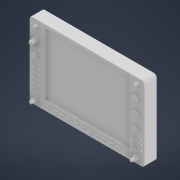
# Autodesk Inventor part: G1000
Saved by Autodesk Inventor 2022 (Build 260153000, 153)
## iProperties
Created: 2022-01-12
Part Number: G1000
Material: Generic
Document SubType Name: Modeling
Designer: diabolous
Density: 1 g/cm^3
Appearance: Default
Author: diabolous
Autodesk Inventor part; units mm, degrees
ref_plane "YZ Plane" through (0, 0, 0) normal (1, 0, 0) x (0, 1, 0)
ref_plane "XZ Plane" through (0, 0, 0) normal (0, 1, 0) x (-1, 0, 0)
ref_plane "XY Plane" through (0, 0, 0) normal (0, 0, 1) x (1, 0, 0)
sketch "Sketch2" plane through (0, 0, 0) normal (0, 0, 1) x (1, 0, 0)
  line L0 (0, 0) -> (296.2402, 0)
  line L1 (296.2402, 0) -> (296.2402, 193.548)
  line L2 (296.2402, 193.548) -> (0, 193.548)
  line L3 (0, 193.548) -> (0, 0)
  dimension "d29" = 296.2402
  dimension "d30" = 193.548
  constraints: 8 end point, 2 parallel, 1 horizontal, 1 perpendicular
  measures "d29" distance of L2.end L1.end
  measures "d30" distance of L1.end L0.end
extrude "Extrusion1" add sketch "Sketch2" along normal blind 32.3
fillet "Fillet1" radius 7.9375 4 edges at (296.2402, 193.548, 16.15) (296.2402, 0, 16.15) (0, 0, 16.15) (0, 193.548, 16.15)
sketch "Sketch3" plane through (0, 0, 32.3) normal (0, 0, 1) x (1, 0, 0)
  line L0 (7.9375, 0) -> (288.3027, 0) projected
  line L1 (296.2402, 7.9375) -> (296.2402, 185.6105) projected
  line L2 (288.3027, 193.548) -> (7.9375, 193.548) projected
  line L3 (0, 185.6105) -> (0, 7.9375) projected
  line L4 (0, 185.6105) -> (0, 7.9375) projected
  line L5 (40.7162, 183.3372) -> (255.524, 183.3372)
  line L6 (255.524, 183.3372) -> (255.524, 22.987)
  line L7 (255.524, 22.987) -> (40.7162, 22.987)
  line L8 (40.7162, 22.987) -> (40.7162, 183.3372)
  point P0 (0, 0)
  point P1 (40.7162, 0)
  point P2 (255.524, 0)
  point P3 (296.2402, 183.3372)
  point P4 (255.524, 193.548)
  point P5 (40.7162, 193.548)
  point P6 (0, 22.987)
  point P7 (296.2402, 22.987)
  point P8 (0, 183.3372)
  dimension "d34" = 40.7162
  dimension "d35" = 40.7162
  dimension "d36" = 10.2108
  dimension "d37" = 40.7162
  dimension "d38" = 22.987
  dimension "d39" = 22.987
  dimension "d40" = 40.7162
  dimension "d41" = 10.2108
  constraints: 8 end point, 6 point on line, 2 parallel, 1 horizontal, 1 perpendicular
  measures "d34" distance of point (40.716, 0) point (0, 0)
  measures "d35" distance from line of L1 point (255.524, 193.548)
  measures "d36" distance from line of L2 point (296.24, 183.337)
  measures "d37" distance from line of L1 point (255.524, 0)
  measures "d38" distance from line of L0 point (296.24, 22.987)
  measures "d39" distance from line of point (0, 22.987) L0
  measures "d40" distance from line of L3 point (40.716, 193.548)
  measures "d41" distance from line of L2 point (0, 183.337)
extrude "Extrusion2" cut sketch "Sketch3" against normal blind 5.08
sketch "Sketch4" plane through (0, 0, 32.3) normal (0, 0, 1) x (1, 0, 0)
  line L0 (288.3027, 193.548) -> (7.9375, 193.548) projected
  line L1 (296.2402, 7.9375) -> (296.2402, 185.6105) projected
  line L2 (0, 185.6105) -> (0, 7.9375) projected
  circle A0 centre (18.5928, 178.5874) radius 3.9243
  circle A1 centre (277.6474, 178.5874) radius 3.9243
  point P0 (0, 0)
  point P1 (0, 178.5874)
  point P2 (18.5928, 193.548)
  point P3 (277.6474, 193.548)
  point P4 (296.2402, 178.5874)
  dimension "d44" = 14.9606
  dimension "d45" = 14.9606
  dimension "d46" = 18.5928
  dimension "d47" = 18.5928
  dimension "d48" = 7.8486
  constraints: 3 point on line, 2 centre point
  measures "d44" distance from line of L0 point (0, 178.587)
  measures "d45" distance from line of L0 point (296.24, 178.587)
  measures "d46" distance from line of L2 point (18.593, 193.548)
  measures "d47" distance from line of L1 point (277.647, 193.548)
  measures "d48" diameter of A0
extrude "Extrusion3" add sketch "Sketch4" along normal blind 8.255
sketch "Sketch5" plane through (0, 0, 32.3) normal (0, 0, 1) x (1, 0, 0)
  circle A0 centre (18.5928, 178.5874) radius 3.9243 projected
  line L0 (18.5928, 178.5874) -> (18.5928, 0) construction
  line L1 (7.9375, 0) -> (288.3027, 0) projected
  line L2 (0, 185.6105) -> (0, 7.9375) projected
  line L3 (288.3027, 193.548) -> (7.9375, 193.548) projected
  circle A1 centre (18.5928, 149.3012) radius 6.1341
  circle A2 centre (18.5928, 115.2144) radius 6.1849
  circle A3 centre (18.5928, 15.9766) radius 6.096
  point P0 (0, 0)
  point P1 (0, 149.3012)
  point P2 (0, 115.2144)
  point P3 (0, 15.9766)
  dimension "d51" = 44.2468
  dimension "d52" = 78.3336
  dimension "d53" = 177.5714
  dimension "d54" = 12.2682
  dimension "d55" = 12.3698
  dimension "d56" = 12.192
  constraints: 7 point on line, 3 centre point, 2 end point, 1 vertical
  measures "d51" distance from line of point (0, 149.301) L3
  measures "d52" distance from line of L3 point (0, 115.214)
  measures "d53" distance from line of L3 point (0, 15.977)
  measures "d54" diameter of A1
  measures "d55" diameter of A2
  measures "d56" diameter of A3
extrude "Extrusion4" add sketch "Sketch5" along normal blind 8.255 contours A1 | A2 | A3
sketch "Sketch6" plane through (18.5928, 115.2144, 40.555) normal (0, 0, 1) x (1, 0, 0)
  circle A0 centre (0, 34.0868) radius 6.1341 projected
  circle A1 centre (0, 34.0868) radius 4.8387
  circle A2 centre (0, -99.2378) radius 6.096 projected
  circle A3 centre (0, -99.2378) radius 3.9751
  point P0 (-18.5928, -115.2144)
  dimension "d59" = 9.6774
  dimension "d60" = 7.9502
  constraints: 2 centre point, 2 coincident
  measures "d59" diameter of A1
  measures "d60" diameter of A3
extrude "Extrusion5" add sketch "Sketch6" along normal blind 8.255 contours A1 | A3
sketch "Sketch7" plane through (0, 0, 32.3) normal (0, 0, 1) x (1, 0, 0)
  line L0 (7.9375, 0) -> (288.3027, 0) projected
  line L1 (40.7162, 11.9126) -> (255.524, 11.9126) construction
  line L2 (148.1201, 0) -> (148.1201, 193.548) construction
  line L3 (288.3027, 193.548) -> (7.9375, 193.548) projected
  line L4 (54.2163, 9.3726) -> (44.0563, 9.3726)
  line L5 (44.0563, 9.3726) -> (44.0563, 14.4526)
  line L6 (44.0563, 14.4526) -> (54.2163, 14.4526)
  line L7 (54.2163, 14.4526) -> (54.2163, 9.3726)
  line L8 (54.2163, 9.3726) -> (44.0563, 14.4526) construction
  line L9 (44.0563, 9.3726) -> (54.2163, 14.4526) construction
  line L10 (72.1487, 9.3726) -> (61.9887, 9.3726)
  line L11 (61.9887, 9.3726) -> (61.9887, 14.4526)
  line L12 (61.9887, 14.4526) -> (72.1487, 14.4526)
  line L13 (72.1487, 14.4526) -> (72.1487, 9.3726)
  line L14 (72.1487, 9.3726) -> (61.9887, 14.4526) construction
  line L15 (61.9887, 9.3726) -> (72.1487, 14.4526) construction
  line L16 (90.0811, 9.3726) -> (79.9211, 9.3726)
  line L17 (79.9211, 9.3726) -> (79.9211, 14.4526)
  line L18 (79.9211, 14.4526) -> (90.0811, 14.4526)
  line L19 (90.0811, 14.4526) -> (90.0811, 9.3726)
  line L20 (90.0811, 9.3726) -> (79.9211, 14.4526) construction
  line L21 (79.9211, 9.3726) -> (90.0811, 14.4526) construction
  line L22 (108.0135, 9.3726) -> (97.8535, 9.3726)
  line L23 (97.8535, 9.3726) -> (97.8535, 14.4526)
  line L24 (97.8535, 14.4526) -> (108.0135, 14.4526)
  line L25 (108.0135, 14.4526) -> (108.0135, 9.3726)
  line L26 (108.0135, 9.3726) -> (97.8535, 14.4526) construction
  line L27 (97.8535, 9.3726) -> (108.0135, 14.4526) construction
  line L28 (125.9459, 9.3726) -> (115.7859, 9.3726)
  line L29 (115.7859, 9.3726) -> (115.7859, 14.4526)
  line L30 (115.7859, 14.4526) -> (125.9459, 14.4526)
  line L31 (125.9459, 14.4526) -> (125.9459, 9.3726)
  line L32 (125.9459, 9.3726) -> (115.7859, 14.4526) construction
  line L33 (115.7859, 9.3726) -> (125.9459, 14.4526) construction
  line L34 (143.8783, 9.3726) -> (133.7183, 9.3726)
  line L35 (133.7183, 9.3726) -> (133.7183, 14.4526)
  line L36 (133.7183, 14.4526) -> (143.8783, 14.4526)
  line L37 (143.8783, 14.4526) -> (143.8783, 9.3726)
  line L38 (143.8783, 9.3726) -> (133.7183, 14.4526) construction
  line L39 (133.7183, 9.3726) -> (143.8783, 14.4526) construction
  line L40 (162.5219, 9.3726) -> (152.3619, 9.3726)
  line L41 (152.3619, 9.3726) -> (152.3619, 14.4526)
  line L42 (152.3619, 14.4526) -> (162.5219, 14.4526)
  line L43 (162.5219, 14.4526) -> (162.5219, 9.3726)
  line L44 (162.5219, 9.3726) -> (152.3619, 14.4526) construction
  line L45 (152.3619, 9.3726) -> (162.5219, 14.4526) construction
  line L46 (180.4543, 9.3726) -> (170.2943, 9.3726)
  line L47 (170.2943, 9.3726) -> (170.2943, 14.4526)
  line L48 (170.2943, 14.4526) -> (180.4543, 14.4526)
  line L49 (180.4543, 14.4526) -> (180.4543, 9.3726)
  line L50 (180.4543, 9.3726) -> (170.2943, 14.4526) construction
  line L51 (170.2943, 9.3726) -> (180.4543, 14.4526) construction
  line L52 (198.3867, 9.3726) -> (188.2267, 9.3726)
  line L53 (188.2267, 9.3726) -> (188.2267, 14.4526)
  line L54 (188.2267, 14.4526) -> (198.3867, 14.4526)
  line L55 (198.3867, 14.4526) -> (198.3867, 9.3726)
  line L56 (198.3867, 9.3726) -> (188.2267, 14.4526) construction
  line L57 (188.2267, 9.3726) -> (198.3867, 14.4526) construction
  line L58 (216.3191, 9.3726) -> (206.1591, 9.3726)
  line L59 (206.1591, 9.3726) -> (206.1591, 14.4526)
  line L60 (206.1591, 14.4526) -> (216.3191, 14.4526)
  line L61 (216.3191, 14.4526) -> (216.3191, 9.3726)
  line L62 (216.3191, 9.3726) -> (206.1591, 14.4526) construction
  line L63 (206.1591, 9.3726) -> (216.3191, 14.4526) construction
  line L64 (234.2515, 9.3726) -> (224.0915, 9.3726)
  line L65 (224.0915, 9.3726) -> (224.0915, 14.4526)
  line L66 (224.0915, 14.4526) -> (234.2515, 14.4526)
  line L67 (234.2515, 14.4526) -> (234.2515, 9.3726)
  line L68 (234.2515, 9.3726) -> (224.0915, 14.4526) construction
  line L69 (224.0915, 9.3726) -> (234.2515, 14.4526) construction
  line L70 (252.1839, 9.3726) -> (242.0239, 9.3726)
  line L71 (242.0239, 9.3726) -> (242.0239, 14.4526)
  line L72 (242.0239, 14.4526) -> (252.1839, 14.4526)
  line L73 (252.1839, 14.4526) -> (252.1839, 9.3726)
  line L74 (252.1839, 9.3726) -> (242.0239, 14.4526) construction
  line L75 (242.0239, 9.3726) -> (252.1839, 14.4526) construction
  point P0 (0, 0)
  point P1 (138.7983, 11.9126)
  point P2 (120.8659, 11.9126)
  point P3 (102.9335, 11.9126)
  point P4 (85.0011, 11.9126)
  point P5 (67.0687, 11.9126)
  point P6 (49.1363, 11.9126)
  point P7 (157.4419, 11.9126)
  point P8 (175.3743, 11.9126)
  point P9 (193.3067, 11.9126)
  point P10 (211.2391, 11.9126)
  point P11 (229.1715, 11.9126)
  point P12 (247.1039, 11.9126)
  dimension "d63" = 11.9126
  dimension "d64" = 11.9126
  dimension "d65" = 9.3218
  dimension "d66" = 17.9324
  dimension "d67" = 17.9324
  dimension "d68" = 17.9324
  dimension "d69" = 17.9324
  dimension "d70" = 17.9324
  dimension "d71" = 9.3218
  dimension "d72" = 17.9324
  dimension "d73" = 17.9324
  dimension "d74" = 17.9324
  dimension "d75" = 17.9324
  dimension "d76" = 17.9324
  dimension "d77" = 10.16
  dimension "d78" = 5.08
  dimension "d79" = 10.16
  dimension "d80" = 10.16
  dimension "d81" = 10.16
  dimension "d82" = 10.16
  dimension "d83" = 10.16
  dimension "d84" = 10.16
  dimension "d85" = 10.16
  dimension "d86" = 10.16
  dimension "d87" = 10.16
  dimension "d88" = 10.16
  dimension "d89" = 10.16
  constraints: 146 end point, 26 midpoint, 24 parallel, 12 horizontal, 12 perpendicular, 11 point on line, 15 other
  measures "d63" distance from line of L0 point (40.716, 11.913)
  measures "d64" distance from line of L0 point (255.524, 11.913)
  measures "d65" distance from line of L2 point (138.798, 11.913)
  measures "d66" distance of point (138.798, 11.913) point (120.866, 11.913)
  measures "d67" distance of point (102.934, 11.913) point (120.866, 11.913)
  measures "d68" distance of point (85.001, 11.913) point (102.934, 11.913)
  measures "d69" distance of point (67.069, 11.913) point (85.001, 11.913)
  measures "d70" distance of point (49.136, 11.913) point (67.069, 11.913)
  measures "d71" distance from line of point (157.442, 11.913) L2
  measures "d72" distance of point (175.374, 11.913) point (157.442, 11.913)
  measures "d73" distance of point (193.307, 11.913) point (175.374, 11.913)
  measures "d74" distance of point (211.239, 11.913) point (193.307, 11.913)
  measures "d75" distance of point (229.172, 11.913) point (211.239, 11.913)
  measures "d76" distance of point (247.104, 11.913) point (229.172, 11.913)
  measures "d77" distance of L5.end L6.end
  measures "d78" distance of L4.end L5.end
  measures "d79" distance of L11.end L12.end
  measures "d80" distance of L17.end L18.end
  measures "d81" distance of L23.end L24.end
  measures "d82" distance of L29.end L30.end
  measures "d83" distance of L35.end L36.end
  measures "d84" distance of L41.end L42.end
  measures "d85" distance of L47.end L48.end
  measures "d86" distance of L53.end L54.end
  measures "d87" distance of L59.end L60.end
  measures "d88" distance of L65.end L66.end
  measures "d89" distance of L71.end L72.end
extrude "Extrusion6" add sketch "Sketch7" along normal blind 1.905
fillet "Fillet2" radius 2.54 1 edges at (14.6685, 178.5874, 32.3)
fillet "Fillet3" radius 2.54 4 edges at (12.4587, 149.3012, 32.3) (12.4079, 115.2144, 32.3) (12.4968, 15.9766, 32.3) (273.7231, 178.5874, 32.3)
fillet "Fillet4" radius 2.54 8 edges at (40.7162, 103.1621, 27.22) (148.1201, 22.987, 27.22) (148.1201, 183.3372, 27.22) (255.524, 103.1621, 27.22) (40.7162, 103.1621, 32.3) (148.1201, 22.987, 32.3) (148.1201, 183.3372, 32.3) (255.524, 103.1621, 32.3)
fillet "Fillet5" radius 0.9525 23 edges at (14.6685, 178.5874, 40.555) (12.4587, 149.3012, 40.555) (13.7541, 149.3012, 48.81) (12.4079, 115.2144, 40.555) (14.6177, 15.9766, 48.81) (12.4968, 15.9766, 40.555) (293.9154, 2.3248, 32.3) (296.2402, 96.774, 32.3) (293.9154, 191.2232, 32.3) (148.1201, 193.548, 32.3) (2.3248, 191.2232, 32.3) (0, 96.774, 32.3) (2.3248, 2.3248, 32.3) (148.1201, 0, 32.3) (273.7231, 178.5874, 40.555) (293.9154, 191.2232, 0) (148.1201, 193.548, 0) (2.3248, 191.2232, 0) (0, 96.774, 0) (2.3248, 2.3248, 0) (148.1201, 0, 0) (293.9154, 2.3248, 0) (296.2402, 96.774, 0)
sketch "Sketch8" plane through (0, 0, 32.3) normal (0, 0, 1) x (1, 0, 0)
  circle A0 centre (277.6474, 178.5874) radius 3.9243 projected
  line L0 (277.6474, 178.5874) -> (277.6474, -3.1455)
  line L1 (288.3027, 193.548) -> (7.9375, 193.548) projected
  circle A1 centre (277.6474, 149.3012) radius 6.1341
  circle A2 centre (277.6474, 115.2144) radius 6.1849
  point P0 (0, 0)
  dimension "d96" = 44.2468
  dimension "d97" = 12.2682
  dimension "d98" = 78.3336
  dimension "d99" = 12.3698
  constraints: 2 centre point, 2 coincident, 2 end point, 2 point on line, 1 vertical
  measures "d96" distance from line of point (277.647, 149.301) L1
  measures "d97" diameter of A1
  measures "d98" distance from line of point (277.647, 115.214) L1
  measures "d99" diameter of A2
extrude "Extrusion7" add sketch "Sketch8" along normal blind 8.255 contours A1 L0 | L0 A1 | A2 L0 | L0 A2
fillet "Fillet6" radius 0.9525 2 edges at (271.5133, 149.3012, 40.555) (271.4625, 115.2144, 40.555)
sketch "Sketch9" plane through (0, 0, 32.3) normal (0, 0, 1) x (1, 0, 0)
  circle A0 centre (18.5928, 15.9766) radius 3.0226 projected
  circle A1 centre (277.6474, 115.2144) radius 5.2324 projected
  circle A2 centre (277.6474, 15.9766) radius 6.096
  point P0 (0, 0)
  dimension "d103" = 12.192
  constraints: 1 centre point
  measures "d103" diameter of A2
extrude "Extrusion8" add sketch "Sketch9" along normal blind 8.255 contours A2
sketch "Sketch10" plane through (277.6474, 15.9766, 40.555) normal (0, 0, 1) x (1, 0, 0)
  circle A0 centre (0, 0) radius 6.096 projected
  circle A1 centre (0, 0) radius 3.9751
  point P0 (-277.6474, -15.9766)
  dimension "d106" = 7.9502
  constraints: 1 centre point, 1 coincident
  measures "d106" diameter of A1
extrude "Extrusion9" add sketch "Sketch10" along normal blind 8.255 contours A1
sketch "Sketch11" plane through (0, 0, 32.3) normal (0, 0, 1) x (1, 0, 0)
  line L0 (296.2402, 7.9375) -> (296.2402, 185.6105) projected
  line L1 (288.3027, 0.9525) -> (7.9375, 0.9525) projected
  line L2 (295.2877, 185.6105) -> (295.2877, 7.9375) projected
  line L3 (7.9375, 0) -> (288.3027, 0) projected
  line L4 (269.9512, 0) -> (269.9512, 58.6486) construction
  line L5 (284.6578, 0.9525) -> (284.6578, 58.6486) construction
  line L6 (284.6578, 35.9918) -> (269.9512, 35.9918) construction
  line L7 (284.6578, 47.3202) -> (269.9512, 47.3202) construction
  line L8 (284.6578, 58.6486) -> (269.9512, 58.6486) construction
  line L9 (264.8712, 38.5318) -> (275.0312, 38.5318)
  line L10 (275.0312, 38.5318) -> (275.0312, 33.4518)
  line L11 (275.0312, 33.4518) -> (264.8712, 33.4518)
  line L12 (264.8712, 33.4518) -> (264.8712, 38.5318)
  line L13 (264.8712, 38.5318) -> (275.0312, 33.4518) construction
  line L14 (275.0312, 38.5318) -> (264.8712, 33.4518) construction
  line L15 (289.7378, 33.4518) -> (279.5778, 33.4518)
  line L16 (279.5778, 33.4518) -> (279.5778, 38.5318)
  line L17 (279.5778, 38.5318) -> (289.7378, 38.5318)
  line L18 (289.7378, 38.5318) -> (289.7378, 33.4518)
  line L19 (289.7378, 33.4518) -> (279.5778, 38.5318) construction
  line L20 (279.5778, 33.4518) -> (289.7378, 38.5318) construction
  line L21 (264.8712, 49.8602) -> (275.0312, 49.8602)
  line L22 (275.0312, 49.8602) -> (275.0312, 44.7802)
  line L23 (275.0312, 44.7802) -> (264.8712, 44.7802)
  line L24 (264.8712, 44.7802) -> (264.8712, 49.8602)
  line L25 (264.8712, 49.8602) -> (275.0312, 44.7802) construction
  line L26 (275.0312, 49.8602) -> (264.8712, 44.7802) construction
  line L27 (289.7378, 44.7802) -> (279.5778, 44.7802)
  line L28 (279.5778, 44.7802) -> (279.5778, 49.8602)
  line L29 (279.5778, 49.8602) -> (289.7378, 49.8602)
  line L30 (289.7378, 49.8602) -> (289.7378, 44.7802)
  line L31 (289.7378, 44.7802) -> (279.5778, 49.8602) construction
  line L32 (279.5778, 44.7802) -> (289.7378, 49.8602) construction
  line L33 (264.8712, 61.1886) -> (275.0312, 61.1886)
  line L34 (275.0312, 61.1886) -> (275.0312, 56.1086)
  line L35 (275.0312, 56.1086) -> (264.8712, 56.1086)
  line L36 (264.8712, 56.1086) -> (264.8712, 61.1886)
  line L37 (264.8712, 61.1886) -> (275.0312, 56.1086) construction
  line L38 (275.0312, 61.1886) -> (264.8712, 56.1086) construction
  line L39 (289.7378, 61.1886) -> (279.5778, 61.1886)
  line L40 (279.5778, 61.1886) -> (279.5778, 56.1086)
  line L41 (279.5778, 56.1086) -> (289.7378, 56.1086)
  line L42 (289.7378, 56.1086) -> (289.7378, 61.1886)
  line L43 (289.7378, 61.1886) -> (279.5778, 56.1086) construction
  line L44 (279.5778, 61.1886) -> (289.7378, 56.1086) construction
  point P0 (0, 0)
  point P1 (295.2877, 35.9918)
  point P2 (295.2877, 47.3202)
  point P3 (295.2877, 58.6486)
  dimension "d109" = 26.289
  dimension "d110" = 11.5824
  dimension "d111" = 35.9918
  dimension "d112" = 47.3202
  dimension "d113" = 58.6486
  dimension "d114" = 10.16
  dimension "d115" = 5.08
  dimension "d116" = 10.16
  dimension "d117" = 5.08
  dimension "d118" = 5.08
  constraints: 82 end point, 15 point on line, 14 parallel, 12 midpoint, 8 perpendicular, 6 horizontal, 1 vertical
  measures "d109" distance from line of L0 L4.start
  measures "d110" distance from line of L0 L5.start
  measures "d111" distance from line of point (295.288, 35.992) L3
  measures "d112" distance from line of L3 point (295.288, 47.32)
  measures "d113" distance from line of point (295.288, 58.649) L3
  measures "d114" distance of L10.end L11.end
  measures "d115" distance of L9.end L10.end
  measures "d116" distance of L16.end L17.end
  measures "d117" distance of L21.end L22.end
  measures "d118" distance of L33.end L34.end
extrude "Extrusion10" add sketch "Sketch11" along normal blind 1.905
sketch "Sketch12" plane through (0, 0, 32.3) normal (0, 0, 1) x (1, 0, 0)
  circle A0 centre (277.6474, 115.2144) radius 5.2324 projected
  line L0 (288.3027, 193.548) -> (7.9375, 193.548) projected
  circle A1 centre (277.6474, 81.788) radius 4.6482
  point P0 (0, 0)
  dimension "d121" = 111.76
  dimension "d122" = 9.2964
  constraints: 1 centre point, 1 coincident
  measures "d121" distance from line of point (277.647, 81.788) L0
  measures "d122" diameter of A1
extrude "Extrusion11" add sketch "Sketch12" along normal blind 8.255 contours A1
fillet "Fillet7" radius 0.9525 1 edges at (272.9992, 81.788, 40.555)
sketch "Sketch13" plane through (0, 0, 32.3) normal (0, 0, 1) x (1, 0, 0)
  line L0 (264.8712, 56.1086) -> (264.8712, 61.1886) projected
  line L1 (0.9525, 7.9375) -> (0.9525, 185.6105) projected
  line L2 (264.8712, 44.7802) -> (264.8712, 49.8602) projected
  line L3 (264.8712, 33.4518) -> (264.8712, 38.5318) projected
  line L4 (288.3027, 0.9525) -> (7.9375, 0.9525) projected
  line L5 (0, 185.6105) -> (0, 7.9375) projected
  line L6 (16.6624, 33.4518) -> (6.5024, 33.4518)
  line L7 (6.5024, 33.4518) -> (6.5024, 38.5318)
  line L8 (6.5024, 38.5318) -> (16.6624, 38.5318)
  line L9 (16.6624, 38.5318) -> (16.6624, 33.4518)
  line L10 (16.6624, 33.4518) -> (6.5024, 38.5318) construction
  line L11 (6.5024, 33.4518) -> (16.6624, 38.5318) construction
  line L12 (31.369, 33.4518) -> (21.209, 33.4518)
  line L13 (21.209, 33.4518) -> (21.209, 38.5318)
  line L14 (21.209, 38.5318) -> (31.369, 38.5318)
  line L15 (31.369, 38.5318) -> (31.369, 33.4518)
  line L16 (31.369, 33.4518) -> (21.209, 38.5318) construction
  line L17 (21.209, 33.4518) -> (31.369, 38.5318) construction
  line L18 (16.6624, 44.7802) -> (6.5024, 44.7802)
  line L19 (6.5024, 44.7802) -> (6.5024, 49.8602)
  line L20 (6.5024, 49.8602) -> (16.6624, 49.8602)
  line L21 (16.6624, 49.8602) -> (16.6624, 44.7802)
  line L22 (16.6624, 44.7802) -> (6.5024, 49.8602) construction
  line L23 (6.5024, 44.7802) -> (16.6624, 49.8602) construction
  line L24 (31.369, 44.7802) -> (21.209, 44.7802)
  line L25 (21.209, 44.7802) -> (21.209, 49.8602)
  line L26 (21.209, 49.8602) -> (31.369, 49.8602)
  line L27 (31.369, 49.8602) -> (31.369, 44.7802)
  line L28 (31.369, 44.7802) -> (21.209, 49.8602) construction
  line L29 (21.209, 44.7802) -> (31.369, 49.8602) construction
  line L30 (16.6624, 56.1086) -> (6.5024, 56.1086)
  line L31 (6.5024, 56.1086) -> (6.5024, 61.1886)
  line L32 (6.5024, 61.1886) -> (16.6624, 61.1886)
  line L33 (16.6624, 61.1886) -> (16.6624, 56.1086)
  line L34 (16.6624, 56.1086) -> (6.5024, 61.1886) construction
  line L35 (6.5024, 56.1086) -> (16.6624, 61.1886) construction
  line L36 (31.369, 56.1086) -> (21.209, 56.1086)
  line L37 (21.209, 56.1086) -> (21.209, 61.1886)
  line L38 (21.209, 61.1886) -> (31.369, 61.1886)
  line L39 (31.369, 61.1886) -> (31.369, 56.1086)
  line L40 (31.369, 56.1086) -> (21.209, 61.1886) construction
  line L41 (21.209, 56.1086) -> (31.369, 61.1886) construction
  line L42 (16.6624, 67.437) -> (6.5024, 67.437)
  line L43 (6.5024, 67.437) -> (6.5024, 72.517)
  line L44 (6.5024, 72.517) -> (16.6624, 72.517)
  line L45 (16.6624, 72.517) -> (16.6624, 67.437)
  line L46 (16.6624, 67.437) -> (6.5024, 72.517) construction
  line L47 (6.5024, 67.437) -> (16.6624, 72.517) construction
  line L48 (31.369, 67.437) -> (21.209, 67.437)
  line L49 (21.209, 67.437) -> (21.209, 72.517)
  line L50 (21.209, 72.517) -> (31.369, 72.517)
  line L51 (31.369, 72.517) -> (31.369, 67.437)
  line L52 (31.369, 67.437) -> (21.209, 72.517) construction
  line L53 (21.209, 67.437) -> (31.369, 72.517) construction
  line L54 (16.6624, 78.7654) -> (6.5024, 78.7654)
  line L55 (6.5024, 78.7654) -> (6.5024, 83.8454)
  line L56 (6.5024, 83.8454) -> (16.6624, 83.8454)
  line L57 (16.6624, 83.8454) -> (16.6624, 78.7654)
  line L58 (16.6624, 78.7654) -> (6.5024, 83.8454) construction
  line L59 (6.5024, 78.7654) -> (16.6624, 83.8454) construction
  line L60 (31.369, 78.7654) -> (21.209, 78.7654)
  line L61 (21.209, 78.7654) -> (21.209, 83.8454)
  line L62 (21.209, 83.8454) -> (31.369, 83.8454)
  line L63 (31.369, 83.8454) -> (31.369, 78.7654)
  line L64 (31.369, 78.7654) -> (21.209, 83.8454) construction
  line L65 (21.209, 78.7654) -> (31.369, 83.8454) construction
  line L66 (16.6624, 90.0938) -> (6.5024, 90.0938)
  line L67 (6.5024, 90.0938) -> (6.5024, 95.1738)
  line L68 (6.5024, 95.1738) -> (16.6624, 95.1738)
  line L69 (16.6624, 95.1738) -> (16.6624, 90.0938)
  line L70 (16.6624, 90.0938) -> (6.5024, 95.1738) construction
  line L71 (6.5024, 90.0938) -> (16.6624, 95.1738) construction
  line L72 (31.369, 90.0938) -> (21.209, 90.0938)
  line L73 (21.209, 90.0938) -> (21.209, 95.1738)
  line L74 (21.209, 95.1738) -> (31.369, 95.1738)
  line L75 (31.369, 95.1738) -> (31.369, 90.0938)
  line L76 (31.369, 90.0938) -> (21.209, 95.1738) construction
  line L77 (21.209, 90.0938) -> (31.369, 95.1738) construction
  point P0 (0, 0)
  point P1 (11.5824, 0.9525)
  point P2 (26.289, 0.9525)
  point P3 (11.5824, 35.9918)
  point P4 (26.289, 35.9918)
  point P5 (11.5824, 47.3202)
  point P6 (26.289, 47.3202)
  point P7 (11.5824, 58.6486)
  point P8 (26.289, 58.6486)
  point P9 (11.5824, 69.977)
  point P10 (26.289, 69.977)
  point P11 (11.5824, 81.3054)
  point P12 (26.289, 81.3054)
  dimension "d126" = 11.5824
  dimension "d127" = 26.289
  dimension "d131" = 10.16
  dimension "d132" = 10.16
  dimension "d133" = 5.08
  dimension "d134" = 5.08
  dimension "d135" = 5.08
  constraints: 144 end point, 24 parallel, 20 midpoint, 17 point on line, 12 horizontal, 12 perpendicular
  measures "d126" distance from line of point (11.582, 0.953) L5
  measures "d127" horizontal distance of point (0, 0) point (26.289, 0.953)
  measures "d131" distance of L7.end L8.end
  measures "d132" distance of L13.end L14.end
  measures "d133" distance of L42.end L43.end
  measures "d134" distance of L54.end L55.end
  measures "d135" distance of L66.end L67.end
extrude "Extrusion12" add sketch "Sketch13" along normal blind 1.905
fillet "Fillet8" radius 0.9525 2 edges at (271.5514, 15.9766, 40.555) (273.6723, 15.9766, 48.81)
equation "\"d35\" = d34"
equation "\"d37\" = d35"
equation "\"d39\" = d38"
equation "\"d40\" = d34"
equation "\"d41\" = d36"
equation "\"d45\" = d44"
equation "\"d47\" = d46"
equation "\"d67\" = d66"
equation "\"d68\" = d67"
equation "\"d69\" = d68"
equation "\"d70\" = d69"
equation "\"d71\" = d65"
equation "\"d72\" = d66"
equation "\"d73\" = d66"
equation "\"d74\" = d66"
equation "\"d75\" = d66"
equation "\"d76\" = d66"
body "Solid1"
